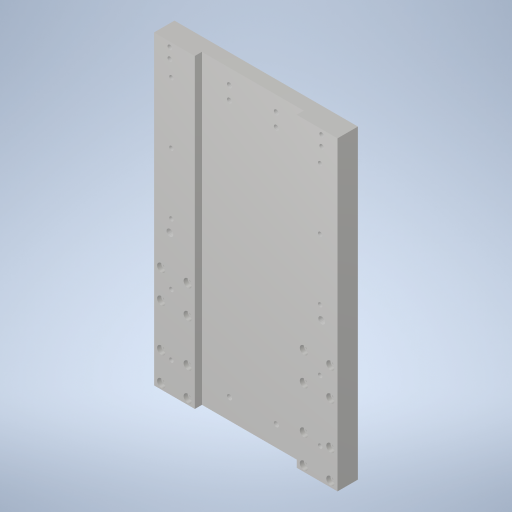
# Autodesk Inventor part: Kreuzplatte
Saved by Autodesk Inventor 2024 (Build 280153020, 153B)
## iProperties
Created: 2021-04-23
Part Number: Kreuzplatte
Material: Aluminium 6061
Document SubType Name: Modeling
Designer: Michael Sumper
Density: 2.7 g/cm^3
Appearance: Aluminium - flach
Mass: 2309.2 g
Surface Area: 1399.25 cm^2
Volume: 855.258 cm^3
Author: Michael Sumper
Autodesk Inventor part; units mm, degrees
ref_plane "YZ Plane" through (0, 0, 0) normal (1, 0, 0) x (0, 1, 0)
ref_plane "XZ Plane" through (0, 0, 0) normal (0, 1, 0) x (-1, 0, 0)
ref_plane "XY Plane" through (0, 0, 0) normal (0, 0, 1) x (1, 0, 0)
sketch "Skizze1" plane through (0, 0, 0) normal (0, 0, 1) x (1, 0, 0)
  line L0 (0, 0) -> (180, 0)
  line L1 (180, 0) -> (180, 300)
  line L2 (180, 300) -> (0, 300)
  line L3 (0, 300) -> (0, 0)
  line L4 (0, 300) -> (17, 300)
  line L5 (17, 300) -> (17, 270)
  line L6 (17, 270) -> (17, 210)
  line L7 (17, 210) -> (17, 150)
  line L8 (17, 150) -> (17, 90)
  line L9 (17, 90) -> (17, 30)
  line L10 (17, 30) -> (17, 0)
  circle A0 centre (17, 270) radius 2.1
  circle A1 centre (17, 210) radius 2.1
  circle A2 centre (17, 150) radius 2.1
  circle A3 centre (17, 90) radius 2.1
  circle A4 centre (17, 30) radius 2.1
  line L11 (0, 300) -> (90, 300)
  line L12 (90, 300) -> (90, 0)
  circle A5 centre (163, 270) radius 2.1
  circle A6 centre (163, 210) radius 2.1
  circle A7 centre (163, 150) radius 2.1
  circle A8 centre (163, 90) radius 2.1
  circle A9 centre (163, 30) radius 2.1
  line L13 (0, 0) -> (0, 5.5)
  line L14 (0, 5.5) -> (35, 5.5)
  line L15 (0, 0) -> (0, 33.5)
  line L16 (0, 33.5) -> (35, 33.5)
  line L17 (0, 0) -> (7, 0)
  line L18 (7, 0) -> (7, 35.5)
  line L19 (0, 0) -> (33, 0)
  line L20 (33, 0) -> (33, 35.5)
  circle A10 centre (7, 5.5) radius 2
  circle A11 centre (33, 5.5) radius 2
  circle A12 centre (33, 33.5) radius 2
  circle A13 centre (7, 33.5) radius 2
  circle A14 centre (173, 5.5) radius 2
  circle A15 centre (147, 5.5) radius 2
  circle A16 centre (147, 33.5) radius 2
  circle A17 centre (173, 33.5) radius 2
  line L21 (17, 300) -> (17, 32.1)
  line L22 (17, 27.9) -> (17, 0)
  line L23 (180, 300) -> (140, 300)
  line L24 (140, 300) -> (140, 0)
  line L25 (0, 300) -> (40, 300)
  line L26 (40, 300) -> (40, 0)
  dimension "d24" = 4
  dimension "d26" = 4
  dimension "d0" = 180
  dimension "d1" = 300
  dimension "d2" = 17
  dimension "d6" = 30
  dimension "d7" = 60
  dimension "d8" = 60
  dimension "d9" = 180
  dimension "d10" = 60
  dimension "d11" = 60
  dimension "d12" = 4.2
  dimension "d13" = 4.2
  dimension "d14" = 4.2
  dimension "d15" = 4.2
  dimension "d16" = 4.2
  dimension "d17" = 90
  dimension "d18" = 300
  dimension "d19" = 5.5
  dimension "d20" = 33.5
  dimension "d21" = 7
  dimension "d22" = 33
  dimension "d23" = 4
  dimension "d25" = 4
  dimension "d27" = 40
  dimension "d28" = 300
  dimension "d29" = 40
  dimension "d30" = 300
  constraints: 54 end point, 21 point on line, 16 centre point, 9 symmetric about line, 5 coincident, 5 perpendicular, 4 point on circle, 2 collinear, 2 midpoint, 2 parallel, 1 horizontal, 1 horizontal alignment, 1 vertical alignment, 13 other
  measures "d0" distance of L2.end L1.end
  measures "d1" distance of L1.end L0.end
  measures "d2" distance of L2.end L4.end
  measures "d6" distance of L4.end L5.end
  measures "d7" distance of L5.end L6.end
  measures "d8" distance of L6.end L7.end
  measures "d9" angle of L7 L6
  measures "d10" distance of L7.end L8.end
  measures "d11" distance of L8.end L9.end
  measures "d12" diameter of A0
  measures "d13" diameter of A1
  measures "d14" diameter of A2
  measures "d15" diameter of A3
  measures "d16" diameter of A4
  measures "d17" distance of L2.end L11.end
  measures "d18" distance of L11.end L12.end
  measures "d19" distance of L0.start L13.end
  measures "d20" distance of L0.start L15.end
  measures "d21" distance of L0.start L17.end
  measures "d22" distance of L0.start L19.end
  measures "d23" diameter of A10
  measures "d25" diameter of A12
  measures "d27" distance of L1.end L23.end
  measures "d28" distance of L23.end L24.end
  measures "d29" distance of L2.end L25.end
  measures "d30" distance of L25.end L26.end
extrude "Extrusion1" add sketch "Skizze1" along normal blind 20
hole "Bohrung1" at (7, 33.5, 0) at (33, 33.5, 0) at (33, 5.5, 0) at (7, 5.5, 0) direction (0, 0, -1) diameter 4 end through all
sketch "Skizze2" plane through (0, 0, 0) normal (0, 0, -1) x (-1, 0, 0)
  circle A0 centre (-33, 33.5) radius 2 projected
  circle A1 centre (-7, 33.5) radius 2 projected
  circle A2 centre (-7, 5.5) radius 2 projected
  circle A3 centre (-33, 5.5) radius 2 projected
  circle A4 centre (-17, 30) radius 2.1 projected
  circle A5 centre (-17, 90) radius 2.1 projected
  circle A6 centre (-17, 150) radius 2.1 projected
  circle A7 centre (-17, 210) radius 2.1 projected
  circle A8 centre (-17, 270) radius 2.1 projected
  point P0 (0, 0)
extrude "Extrusion2" cut sketch "Skizze2" against normal blind 20
sketch "Skizze3" plane through (0, 300, 0) normal (0, 1, 0) x (1, 0, 0)
  line L0 (0, -20) -> (40, -20)
  line L1 (180, -20) -> (0, -20) projected
  line L2 (40, -20) -> (40, -13)
  line L3 (40, -13) -> (140, -13)
  line L4 (140, -13) -> (140, -20)
  line L5 (140, -20) -> (40, -20)
  point P0 (0, 0)
  dimension "d42" = 40
  dimension "d43" = 7
  dimension "d44" = 100
  constraints: 10 end point, 3 perpendicular, 2 point on line, 1 collinear
  measures "d42" distance of L0.start L0.end
  measures "d43" distance of L0.end L2.end
  measures "d44" distance of L2.end L3.end
extrude "Extrusion3" cut sketch "Skizze3" against normal blind 300
sketch "Skizze4" plane through (0, 0, 20) normal (0, 0, 1) x (1, 0, 0)
  circle A0 centre (7, 33.5) radius 2 projected
  circle A1 centre (7, 5.5) radius 2 projected
  line L0 (7, 33.5) -> (7, 5.5)
  line L1 (7, 19.5) -> (7, 89.5)
  line L2 (180, 0) -> (180, 300) projected
  line L3 (7, 54.5) -> (180, 54.5)
  circle A2 centre (33, 33.5) radius 2 projected
  circle A3 centre (33, 5.5) radius 2 projected
  circle A4 centre (7, 5.5) radius 2 projected
  circle A5 centre (147, 33.5) radius 2 projected
  circle A6 centre (147, 5.5) radius 2 projected
  circle A7 centre (173, 33.5) radius 2 projected
  circle A8 centre (173, 5.5) radius 2 projected
  circle A9 centre (7, 75.5) radius 2
  circle A10 centre (7, 103.5) radius 2
  circle A11 centre (33, 75.5) radius 2
  circle A12 centre (33, 103.5) radius 2
  circle A13 centre (147, 75.5) radius 2
  circle A14 centre (147, 103.5) radius 2
  circle A15 centre (173, 75.5) radius 2
  circle A16 centre (173, 103.5) radius 2
  point P0 (0, 0)
  dimension "d67" = 70
  constraints: 8 centre point, 8 symmetric about line, 6 end point, 2 midpoint, 2 point on line, 1 vertical, 8 other
  measures "d67" distance of L1.start L1.end
extrude "Extrusion4" cut sketch "Skizze4" against normal blind 20 contours A9 L1 | L1 A9 | A10 | A11 | A12 | A13 | A14 | A15 | A16
sketch "Skizze5" plane through (0, 0, 20) normal (0, 0, 1) x (1, 0, 0)
  circle A0 centre (7, 33.5) radius 2 projected
  circle A1 centre (33, 33.5) radius 2 projected
  circle A2 centre (7, 5.5) radius 2 projected
  circle A3 centre (33, 5.5) radius 2 projected
  circle A4 centre (147, 33.5) radius 2 projected
  circle A5 centre (147, 5.5) radius 2 projected
  circle A6 centre (173, 5.5) radius 2 projected
  circle A7 centre (173, 33.5) radius 2 projected
  circle A8 centre (173, 75.5) radius 2 projected
  circle A9 centre (147, 75.5) radius 2 projected
  circle A10 centre (33, 75.5) radius 2 projected
  circle A11 centre (7, 75.5) radius 2 projected
  circle A12 centre (33, 103.5) radius 2 projected
  circle A13 centre (7, 103.5) radius 2 projected
  circle A14 centre (147, 103.5) radius 2 projected
  circle A15 centre (173, 103.5) radius 2 projected
  point P0 (0, 0)
hole "Bohrung2" at (7, 103.5, 20) at (33, 103.5, 20) at (7, 75.5, 20) at (33, 75.5, 20) at (7, 33.5, 20) at (33, 33.5, 20) at (33, 5.5, 20) at (7, 5.5, 20) at (147, 75.5, 20) at (173, 75.5, 20) at (173, 33.5, 20) at (147, 33.5, 20) at (147, 103.5, 20) at (173, 103.5, 20) at (147, 5.5, 20) at (173, 5.5, 20) direction (0, 0, -1) diameter 4.8 end through all counterbore diameter 8 counterbore depth 4 clearance for "Innensechskantkopfschraube" size "M4" standard "ANSI Metrisches M Profil"
sketch "Skizze6" plane through (40, 300, 13) normal (0, 0, 1) x (1, 0, 0)
  line L0 (50, 0) -> (73, 0) construction
  line L1 (73, 0) -> (73, -15) construction
  line L2 (73, -15) -> (27, -15) construction
  line L3 (73, -15) -> (73, -28) construction
  line L4 (73, -28) -> (27, -28) construction
  line L5 (73, -15) -> (73, -280) construction
  line L6 (73, -280) -> (27, -280) construction
  dimension "d117" = 23
  dimension "d121" = 15
  dimension "d122" = 46
  dimension "d123" = 13
  dimension "d124" = 46
  dimension "d125" = 265
  dimension "d134" = 46
  constraints: 14 end point, 2 horizontal, 1 other
  measures "d117" distance of L0.start L0.end
  measures "d121" distance of L0.end L1.end
  measures "d122" distance of L1.end L2.end
  measures "d123" distance of L1.end L3.end
  measures "d124" distance of L3.end L4.end
  measures "d125" distance of L1.end L5.end
  measures "d134" distance of L5.end L6.end
extrude "Extrusion5" [suppressed]
sketch "Skizze9" plane through (0, 0, 20) normal (0, 0, 1) x (1, 0, 0)
  point P0 (164.4943, 295)
  point P1 (15.5057, 295)
  point P2 (15.5057, 285)
  point P3 (164.4943, 285)
hole "Bohrung6" at (164.4943, 295, 20) at (15.5057, 295, 20) at (15.5057, 285, 20) at (164.4943, 285, 20) direction (0, 0, -1) diameter 4.5 depth 20
sketch "Skizze10" plane through (0, 0, 20) normal (0, 0, 1) x (1, 0, 0)
  point P0 (164.452, 137.4957)
  point P1 (15.5471, 137.4965)
hole "Bohrung8" at (164.452, 137.4957, 20) at (15.5471, 137.4965, 20) direction (0, 0, -1) diameter 6.6 depth 20
hole "Bohrung10" at (67, 285, 13) at (67, 272, 13) at (113, 285, 13) at (113, 272, 13) at (113, 20, 13) at (67, 20, 13) direction (0, 0, -1) diameter 4.917 end through all thread size "M6x1" class "6H" standard "ANSI Metric M Profile"
thread "Gewinde13" size "M4x0.7" class "6H" standard "ISO Metric profile" full length
thread "Gewinde14" size "M4x0.7" class "6H" standard "ISO Metric profile" full length
thread "Gewinde15" size "M4x0.7" class "6H" standard "ISO Metric profile" full length
thread "Gewinde16" size "M4x0.7" class "6H" standard "ISO Metric profile" full length
thread "Gewinde17" size "M4x0.7" class "6H" standard "ISO Metric profile" full length
thread "Gewinde18" size "M4x0.7" class "6H" standard "ISO Metric profile" full length
thread "Gewinde19" size "M4x0.7" class "6H" standard "ISO Metric profile" full length
thread "Gewinde20" size "M4x0.7" class "6H" standard "ISO Metric profile" full length
thread "Gewinde21" size "M4x0.7" class "6H" standard "ISO Metric profile" full length
thread "Gewinde22" size "M4x0.7" class "6H" standard "ISO Metric profile" full length
thread "Gewinde23" size "M6x1" class "6H" standard "ISO Metric profile" full length
thread "Gewinde24" size "M6x1" class "6H" standard "ISO Metric profile" full length
thread "Gewinde25" size "M4x0.7" class "6H" standard "ISO Metric profile" full length
thread "Gewinde26" size "M4x0.7" class "6H" standard "ISO Metric profile" full length
thread "Gewinde27" size "M4x0.7" class "6H" standard "ISO Metric profile" full length
thread "Gewinde28" size "M4x0.7" class "6H" standard "ISO Metric profile" full length
ref_plane "Arbeitsebene1" through (0, 0, 25) normal (0, 0, 1) x (1, 0, 0)
